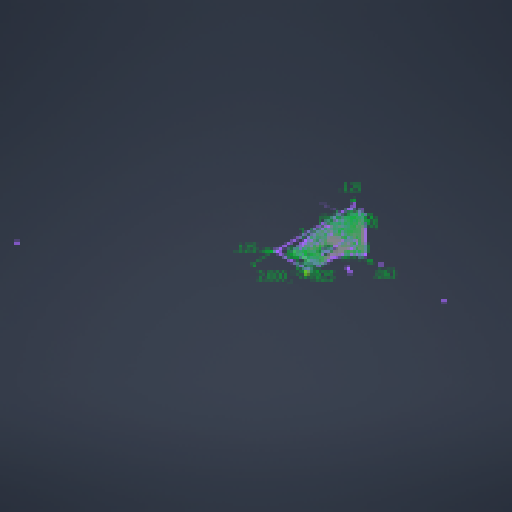
# Autodesk Inventor part: sled2
Saved by Autodesk Inventor 2024 (Build 280153000, 153)
## iProperties
Created: 2023-10-30
Part Number: sled2
Material: Polycarbonate, Smoke
Document SubType Name: Modeling
Designer: macbook
Density: 1.2 g/cm^3
Appearance: Polycarbonate - Clear(1)
Author: macbook
Autodesk Inventor part; units mm, degrees
ref_plane "YZ Plane" through (0, 0, 0) normal (1, 0, 0) x (0, 1, 0)
ref_plane "XZ Plane" through (0, 0, 0) normal (0, 1, 0) x (-1, 0, 0)
ref_plane "XY Plane" through (0, 0, 0) normal (0, 0, 1) x (1, 0, 0)
sketch "Sketch2" plane through (0, 0, 0) normal (0, 1, 0) x (-1, 0, 0)
  line L0 (50.8978, -88.9331) -> (25.3484, -88.9331)
  line L1 (25.3484, -88.9331) -> (25.3484, -76.2331)
  line L2 (25.3484, -76.2331) -> (0.0063, -76.2331)
  line L3 (50.8978, -88.9331) -> (50.8978, -113.4067)
  line L4 (0.0063, -76.2331) -> (0.0055, -63.5331)
  line L5 (0.0055, -63.5331) -> (-22.2195, -63.5346)
  arc A0 (-20.3669, -62.9196) -> (-2.754, -47.4243) centre (-31.4849, -32.5245) ccw
  arc A1 (48.1058, -116.5585) -> (50.8978, -113.4067) centre (47.7228, -113.4067) ccw
  arc A2 (-20.3669, -62.9196) -> (-20.967, -65.5097) centre (-19.8216, -64.4105) ccw
  arc A3 (-2.754, -47.4243) -> (0.0978, -35.7707) centre (-25.3022, -35.7309) ccw
  line L6 (0.0978, -4.698) -> (47.7219, -4.6852)
  line L7 (50.8978, -7.8602) -> (50.8978, -88.9331)
  line L8 (0.0978, -20.5717) -> (0.0978, -35.7707)
  line L9 (3.2719, -4.6971) -> (12.7978, -4.6946)
  line L10 (12.7978, -4.6946) -> (12.8012, -17.3967)
  line L11 (12.8012, -17.3967) -> (20.9, -17.3945)
  line L12 (38.2012, -17.3899) -> (38.2012, -93.5899)
  line L13 (12.8012, -17.3967) -> (12.8012, -68.1967)
  arc A4 (50.8978, -7.8602) -> (47.7219, -4.6852) centre (47.7228, -7.8602) ccw
  arc A5 (3.2719, -4.6971) -> (0.0978, -7.8721) centre (3.2728, -7.8721) ccw
  line L14 (12.8012, -68.1967) -> (12.8012, -74.5467)
  line L15 (38.2012, -93.5899) -> (38.2012, -99.9399)
  line L16 (38.2012, -17.3899) -> (38.2012, -23.7399)
  line L17 (12.8012, -17.3967) -> (12.8012, -23.7467)
  line L18 (12.8012, -23.7467) -> (19.1512, -23.7467)
  line L19 (19.1512, -23.7467) -> (6.4512, -23.7467)
  line L20 (25.3484, -88.9331) -> (31.6984, -88.9331)
  line L21 (31.6984, -88.9331) -> (31.6984, -114.3331)
  arc A6 (-20.967, -65.5097) -> (31.6984, -114.3331) centre (249.7999, 173.7477) ccw
  arc A7 (31.6984, -114.3331) -> (33.1489, -115.4256) centre (249.7999, 173.7477) ccw
  line L22 (38.2012, -88.9331) -> (38.2012, -69.8831)
  line L23 (38.2012, -69.8831) -> (44.7036, -69.8831)
  line L24 (38.2012, -17.3899) -> (16.8506, -17.3956)
  line L25 (12.8012, -17.3967) -> (3.2728, -17.3967)
  arc A8 (38.2012, -113.7028) -> (38.2012, -17.3899) centre (-135.4238, -65.5464) ccw
  arc A9 (33.1489, -115.4256) -> (38.2012, -113.7028) centre (35.0868, -112.839) ccw
  arc A10 (3.2728, -17.3967) -> (0.0978, -20.5717) centre (3.2728, -20.5717) ccw
  line L26 (38.2012, -17.3899) -> (16.8506, -17.3956)
  arc A11 (44.7558, -65.5464) -> (30.4886, -17.392) centre (-43.6427, -65.5464) ccw
  arc A12 (38.2012, -32.1417) -> (24.6857, -17.3935) centre (11.5084, -43.0364) ccw
  arc A13 (32.7636, -23.5578) -> (27.4631, -19.2197) centre (15.0605, -39.7812) ccw
  arc A14 (27.4631, -19.2197) -> (20.9, -17.3945) centre (20.9035, -30.0945) ccw
  line L27 (0.0978, -20.5717) -> (31.8478, -20.5717)
  line L28 (31.8478, -20.5717) -> (31.8478, -76.2331)
  line L29 (31.8478, -17.3916) -> (31.8478, -74.5467)
  line L30 (31.8478, -74.5467) -> (31.6984, -99.9463)
  line L31 (31.6984, -99.9463) -> (31.5861, -119.0417)
  line L32 (31.6984, -99.9463) -> (31.6984, -49.1463)
  line L33 (31.6984, -99.9463) -> (82.4984, -99.9463) construction
  line L34 (31.6984, -49.1463) -> (33.0954, -49.1463)
  line L35 (31.6984, -99.9463) -> (33.0954, -99.9463)
  point P0 (0, 0)
  point P1 (50.8978, -120.6831)
  point P2 (0.0775, -39.6857)
  point P3 (-21.1455, -63.5345)
  point P4 (50.8978, -4.6844)
  point P5 (3.2719, -4.6971)
  point P6 (38.0838, -119.0579)
  point P7 (23.7439, -17.3938)
  point P8 (12.8012, -17.3967)
  dimension "d3" = 12.7
  dimension "d4" = 31.75
  dimension "d5" = 12.7
  dimension "d6" = 22.225
  dimension "d18" = 3.175
  dimension "d19" = 1.5875
  dimension "d23" = 4.699
  dimension "d24" = 12.7
  dimension "d25" = 25.4
  dimension "d26" = 76.2
  dimension "d27" = 50.8
  dimension "d28" = 3.175
  dimension "d33" = 6.35
  dimension "d35" = 6.35
  dimension "d36" = 6.35
  dimension "d37" = 6.35
  dimension "d38" = 12.7
  dimension "d54" = 6.35
  dimension "d55" = 25.4
  dimension "d56" = 50.8
  dimension "d58" = 19.05
  dimension "d59" = 3.175
  dimension "d60" = 12.7
  dimension "d61" = 31.75
  dimension "d62" = 25.4
  dimension "d63" = 19.0957
  dimension "d64" = 180
  dimension "d65" = 50.8
  dimension "d66" = 90
  dimension "d69" = 1.397
  constraints: 72 end point, 39 point on circle, 24 point on line, 16 tangent, 15 centre point, 10 perpendicular, 6 coincident, 6 vertical, 4 horizontal, 3 parallel, 2 collinear, 2 equal radius, 1 midpoint, 1 other
  measures "d3" distance of L0.end L1.end
  measures "d4" distance of L0.start point (50.898, -120.683)
  measures "d5" distance of L2.end L4.end
  measures "d6" distance of L4.end L5.end
  measures "d18" radius of A1
  measures "d19" radius of A2
  measures "d23" distance of point (0, 0) L6.start
  measures "d24" distance of L6.start L9.end
  measures "d25" distance of L10.end L12.start
  measures "d26" distance of L12.start L12.end
  measures "d27" distance of L10.end L13.end
  measures "d28" radius of A4
  measures "d33" distance of L14.start L14.end
  measures "d35" distance of L16.start L16.end
  measures "d36" distance of L17.start L17.end
  measures "d37" distance of L17.end L18.end
  measures "d38" distance of L18.end L19.end
  measures "d54" distance of L0.end L20.end
  measures "d55" distance of L20.end L21.end
  measures "d56" distance between parallel lines of L7 L8
  measures "d58" distance of L22.start L22.end
  measures "d59" radius of A10
  measures "d60" radius of A14
  measures "d61" distance of L8.start L27.end
  measures "d62" distance of L29.end L30.end
  measures "d63" distance of L30.end L31.end
  measures "d64" angle of L31 L30
  measures "d65" distance of L32.start L32.end
  measures "d66" angle of L33 L32
  measures "d69" distance of L34.start L34.end
extrude "Extrusion1" add sketch "Sketch2" along normal blind 1.5875 contours L21 L31 A6 A2 L5 L4 L2 L1 L0 | L32 L34 L28 L30 L0 | L0 L30 L21 | L0 L1 L2 L4 L5 A2 A0 A3 L8 L27 A13 L28 L34 L32 | L30 L28 A12 L12 L0 | L0 A8 A9 A7 L21 L30 | L21 A6 L31 | L12 L23 A8 L0 | L12 A11 A8 L23 | L27 L13 L11 A14 A13 | L27 A10 L25 L13
hole "Hole3" at (-6.4512, 0, -23.7467) at (-19.1512, 0, -23.7467) at (-12.8012, 0, -68.1967) at (-33.0954, 0, -49.1463) at (-33.0954, 0, -99.9463) direction (0, 1, 0) diameter 4.7625 end through all
sketch "Sketch3" plane through (0, 1.5875, 0) normal (0, 1, 0) x (1, 0, 0)
  circle A0 centre (-19.1512, 23.7467) radius 2.3813 projected
  line L0 (-19.1512, 23.7467) -> (-19.1512, 42.7967) construction
  line L1 (-19.1512, 23.7467) -> (-0.1012, 23.7467) construction
  line L2 (-19.1512, 42.7967) -> (-12.8012, 42.7967)
  circle A1 centre (-6.4512, 23.7467) radius 2.3813 projected
  line L3 (-6.4512, 23.7467) -> (-6.4512, 36.4467) construction
  line L4 (-6.4512, 36.4467) -> (-19.1512, 36.4467) construction
  arc A2 (-19.1512, 38.828) -> (-19.1512, 34.0655) centre (-19.1512, 36.4467) ccw
  arc A3 (-6.4512, 34.0655) -> (-6.4512, 38.828) centre (-6.4512, 36.4467) ccw
  line L5 (-19.1512, 34.0655) -> (-6.4512, 34.0655)
  line L6 (-6.4512, 36.4467) -> (-6.4512, 49.1467) construction
  line L7 (-6.4512, 49.1467) -> (-19.1512, 49.1467) construction
  arc A4 (-19.1512, 51.528) -> (-19.1512, 46.7655) centre (-19.1512, 49.1467) ccw
  arc A5 (-6.4512, 46.7655) -> (-6.4512, 51.528) centre (-6.4512, 49.1467) ccw
  line L8 (-6.4512, 51.528) -> (-19.1512, 51.528)
  line L9 (-12.8012, 34.0655) -> (-12.8012, 36.4467)
  line L10 (-12.8012, 36.4467) -> (-19.1512, 36.4467)
  line L11 (-19.1512, 38.828) -> (-15.9722, 38.828)
  line L12 (-6.4512, 38.828) -> (-9.6302, 38.828)
  line L13 (-6.4512, 46.7655) -> (-9.1999, 46.7655)
  line L14 (-19.1512, 46.7655) -> (-16.4024, 46.7655)
  arc A6 (-9.7971, 39.2979) -> (-9.3895, 46.3163) centre (-12.8012, 42.9934) ccw
  arc A7 (-16.2129, 46.3163) -> (-15.8053, 39.2979) centre (-12.8012, 42.9934) ccw
  arc A8 (-9.7971, 39.2979) -> (-9.6302, 38.828) centre (-9.6302, 39.0926) ccw
  arc A9 (-15.9722, 38.828) -> (-15.8053, 39.2979) centre (-15.9722, 39.0926) ccw
  arc A10 (-16.2129, 46.3163) -> (-16.4024, 46.7655) centre (-16.4024, 46.5009) ccw
  arc A11 (-9.1999, 46.7655) -> (-9.3895, 46.3163) centre (-9.1999, 46.5009) ccw
  point P0 (0, 0)
  point P1 (-15.1101, 38.828)
  point P2 (-10.4923, 38.828)
  point P3 (-9.8938, 46.7655)
  point P4 (-15.7085, 46.7655)
  dimension "d70" = 19.05
  dimension "d71" = 90
  dimension "d72" = 6.35
  dimension "d73" = 12.7
  dimension "d78" = 6.35
  dimension "d79" = 0.2646
  constraints: 30 end point, 24 point on circle, 11 point on line, 10 centre point, 10 tangent, 4 coincident, 4 perpendicular, 3 equal radius, 3 vertical, 2 horizontal, 2 midpoint, 1 collinear, 1 parallel
  measures "d70" distance of L0.start L0.end
  measures "d71" angle of L1 L0
  measures "d72" distance of L0.end L2.end
  measures "d73" distance of L3.start L3.end
  measures "d78" distance of L9.end L10.end
  measures "d79" radius of A8
extrude "Extrusion2" cut sketch "Sketch3" against normal through all contours L11 A9 A7 A10 L14 A4 L8 A5 L13 A11 A6 A8 L12 A3 L5 A2
body "Solid1"
